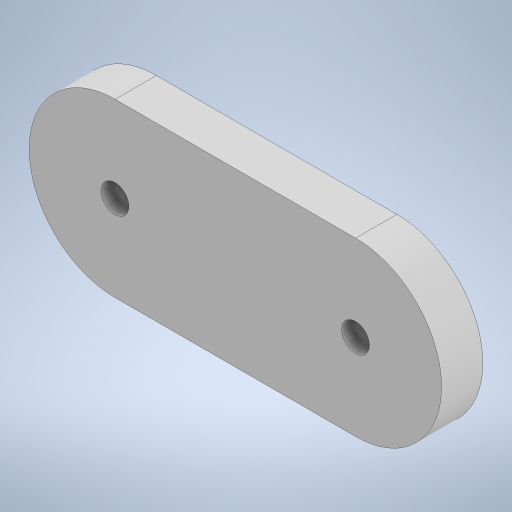
# Autodesk Inventor part: Middle
Saved by Autodesk Inventor 2024 (Build 280153000, 153)
## iProperties
Created: 2024-03-13
Part Number: Middle
Material: Generic
Document SubType Name: Modeling
Designer: ddcos
Density: 1 g/cm^3
Appearance: Default
Author: ddcos
Autodesk Inventor part; units mm, degrees
ref_plane "YZ Plane" through (0, 0, 0) normal (1, 0, 0) x (0, 1, 0)
ref_plane "XZ Plane" through (0, 0, 0) normal (0, 1, 0) x (-1, 0, 0)
ref_plane "XY Plane" through (0, 0, 0) normal (0, 0, 1) x (1, 0, 0)
sketch "Sketch1" plane through (0, 0, 0) normal (0, 0, 1) x (1, 0, 0)
  line L0 (0, 0) -> (-60, 0)
  line L1 (-60, 0) -> (-60, 25)
  line L2 (-60, 25) -> (0, 25)
  line L3 (0, 25) -> (0, 0)
  dimension "d0" = 60
  dimension "d1" = 25
  constraints: 8 end point, 2 parallel, 1 horizontal, 1 perpendicular
  measures "d0" distance of L1.end L2.end
  measures "d1" distance of L2.end L0.start
extrude "Extrusion3" add sketch "Sketch1" along normal blind 6
sketch "Sketch3" plane through (0, 0, 6) normal (0, 0, 1) x (1, 0, 0)
  circle A0 centre (-47.5, 12.5) radius 12.5
  line L0 (-60, 0) -> (0, 0) projected
  line L1 (-60, 25) -> (-60, 0) projected
  circle A1 centre (-12.5, 12.5) radius 12.5
  line L2 (0, 25) -> (-60, 25) projected
  line L3 (0, 0) -> (0, 25) projected
  circle A2 centre (-47.5, 12.5) radius 2
  circle A3 centre (-12.5, 12.5) radius 2
  point P0 (0, 12.5)
  point P1 (-12.5, 0)
  point P2 (-12.5, 25)
  point P3 (-47.5, 25)
  point P4 (-60, 12.5)
  point P5 (-47.5, 0)
  dimension "d16" = 25
  dimension "d17" = 12.5
  dimension "d18" = 12.5
  dimension "d19" = 25
  dimension "d20" = 12.5
  dimension "d21" = 12.5
  dimension "d22" = 4
  dimension "d23" = 4
  constraints: 4 centre point, 2 coincident
  measures "d16" diameter of A0
  measures "d17" distance from line of L0 A0.centre
  measures "d18" distance from line of L1 A0.centre
  measures "d19" diameter of A1
  measures "d20" distance from line of L2 A1.centre
  measures "d21" distance from line of L3 A1.centre
  measures "d22" diameter of A2
  measures "d23" diameter of A3
extrude "Extrusion4" cut sketch "Sketch3" against normal blind 6 contours A0 L1 L2 | L0 L1 A0 | L2 L3 A1 | A1 L3 L0 | A2 | A3
body "Solid2"
